Autodesk Inventor part; units mm, degrees
(part 2 of 3)
sketch "Sketch13" plane through (-0.8, 28.2953, 9.6805) normal (0, 0.9365, 0.3507) x (1, 0, 0)
  line L0 (7.3602, 4.8237) -> (7.6197, 4.2211)
  line L1 (7.6197, 4.2211) -> (8.1859, 3.5794)
  line L2 (8.1859, 3.5794) -> (8.8268, 3.0007)
  line L3 (8.8268, 3.0007) -> (9.6093, 2.8387)
  line L4 (9.6093, 2.8387) -> (10.0903, 2.8061)
  line L5 (10.0903, 2.8061) -> (10.4338, 2.9248)
  line L6 (10.4338, 2.9248) -> (11.3689, 4.0829)
  line L7 (11.3689, 4.0829) -> (11.8797, 4.8558)
  line L8 (11.8797, 4.8558) -> (11.9532, 5.0934)
  line L9 (11.9532, 5.0934) -> (11.8798, 5.2528)
  line L10 (11.8798, 5.2528) -> (11.2166, 5.399)
  line L11 (11.2166, 5.399) -> (9.737, 5.4199)
  line L12 (9.737, 5.4199) -> (7.501, 5.3454)
  line L13 (7.501, 5.3454) -> (7.2801, 5.1684)
  line L14 (7.2801, 5.1684) -> (7.3602, 4.8237)
  line L15 (-11.3774, 3.4883) -> (-9.8778, 1.8277)
  line L16 (-9.8778, 1.8277) -> (-9.5845, 1.6866)
  line L17 (-9.5845, 1.6866) -> (-9.3408, 1.793)
  line L18 (-9.3408, 1.793) -> (-8.9771, 2.2117)
  line L19 (-8.9771, 2.2117) -> (-8.6904, 3.7246)
  line L20 (-8.6904, 3.7246) -> (-8.5682, 4.7047)
  line L21 (-8.5682, 4.7047) -> (-8.7396, 5.208)
  line L22 (-8.7396, 5.208) -> (-9.3955, 5.3934)
  line L23 (-9.3955, 5.3934) -> (-10.727, 5.4199)
  line L24 (-10.727, 5.4199) -> (-12.0368, 5.3897)
  line L25 (-12.0368, 5.3897) -> (-12.5412, 5.1784)
  line L26 (-12.5412, 5.1784) -> (-12.301, 4.605)
  line L27 (-12.301, 4.605) -> (-11.3774, 3.4883)
  line L28 (-0.3781, 3.9581) -> (-0.2709, 2.6186)
  line L29 (-0.2709, 2.6186) -> (0.2264, 2.0123)
  line L30 (0.2264, 2.0123) -> (0.7973, 1.6169)
  line L31 (0.7973, 1.6169) -> (1.4201, 1.7538)
  line L32 (1.4201, 1.7538) -> (1.7893, 1.9111)
  line L33 (1.7893, 1.9111) -> (2.0057, 2.1663)
  line L34 (2.0057, 2.1663) -> (2.3158, 3.6997)
  line L35 (2.3158, 3.6997) -> (2.4451, 4.6942)
  line L36 (2.4451, 4.6942) -> (2.3595, 5.2048)
  line L37 (2.3595, 5.2048) -> (1.9431, 5.393)
  line L38 (1.9431, 5.393) -> (1.0799, 5.4199)
  line L39 (1.0799, 5.4199) -> (0.2133, 5.397)
  line L40 (0.2133, 5.397) -> (-0.2274, 5.2372)
  line L41 (-0.2274, 5.2372) -> (-0.379, 4.8032)
  line L42 (-0.379, 4.8032) -> (-0.3781, 3.9581)
  line L43 (-3.9904, 3.904) -> (-3.9296, 3.009)
  line L44 (-3.9296, 3.009) -> (-3.6926, 2.5158)
  line L45 (-3.6926, 2.5158) -> (-3.1853, 2.3017)
  line L46 (-3.1853, 2.3017) -> (-2.3139, 2.2441)
  line L47 (-2.3139, 2.2441) -> (-1.0191, 2.238)
  line L48 (-1.0191, 2.238) -> (-0.6342, 2.358)
  line L49 (-0.6342, 2.358) -> (-0.4353, 2.664)
  line L50 (-0.4353, 2.664) -> (-0.443, 3.9595)
  line L51 (-0.443, 3.9595) -> (-0.4947, 4.8038)
  line L52 (-0.4947, 4.8038) -> (-0.6992, 5.2373)
  line L53 (-0.6992, 5.2373) -> (-1.2249, 5.3971)
  line L54 (-1.2249, 5.3971) -> (-2.2403, 5.4199)
  line L55 (-2.2403, 5.4199) -> (-3.255, 5.3962)
  line L56 (-3.255, 5.3962) -> (-3.7756, 5.2304)
  line L57 (-3.7756, 5.2304) -> (-3.966, 4.7804)
  line L58 (-3.966, 4.7804) -> (-3.9904, 3.904)
  line L59 (-6.7128, 3.5805) -> (-6.6626, 2.522)
  line L60 (-6.6626, 2.522) -> (-6.5055, 2.0099)
  line L61 (-6.5055, 2.0099) -> (-6.1154, 1.9008)
  line L62 (-6.1154, 1.9008) -> (-5.3661, 2.0514)
  line L63 (-5.3661, 2.0514) -> (-4.6053, 2.2664)
  line L64 (-4.6053, 2.2664) -> (-4.2151, 2.5307)
  line L65 (-4.2151, 2.5307) -> (-4.0727, 3.0178)
  line L66 (-4.0727, 3.0178) -> (-4.0552, 3.901)
  line L67 (-4.0552, 3.901) -> (-4.0794, 4.7791)
  line L68 (-4.0794, 4.7791) -> (-4.2288, 5.23)
  line L69 (-4.2288, 5.23) -> (-4.6308, 5.3961)
  line L70 (-4.6308, 5.3961) -> (-5.4126, 5.4199)
  line L71 (-5.4126, 5.4199) -> (-6.1936, 5.3911)
  line L72 (-6.1936, 5.3911) -> (-6.5893, 5.19)
  line L73 (-6.5893, 5.19) -> (-6.7218, 4.6439)
  line L74 (-6.7218, 4.6439) -> (-6.7128, 3.5805)
  line L75 (-7.9017, 1.7773) -> (-7.0187, 1.5649)
  line L76 (-7.0187, 1.5649) -> (-6.8152, 1.6168)
  line L77 (-6.8152, 1.6168) -> (-6.7773, 3.5664)
  line L78 (-6.7773, 3.5664) -> (-6.9182, 5.1882)
  line L79 (-6.9182, 5.1882) -> (-7.1497, 5.3909)
  line L80 (-7.1497, 5.3909) -> (-7.5903, 5.4199)
  line L81 (-7.5903, 5.4199) -> (-8.0343, 5.3934)
  line L82 (-8.0343, 5.3934) -> (-8.29, 5.2082)
  line L83 (-8.29, 5.2082) -> (-8.6244, 3.7268)
  line L84 (-8.6244, 3.7268) -> (-8.767, 2.744)
  line L85 (-8.767, 2.744) -> (-8.7392, 2.2133)
  line L86 (-8.7392, 2.2133) -> (-8.4734, 1.952)
  line L87 (-8.4734, 1.952) -> (-7.9017, 1.7773)
  line L88 (3.0749, 1.6173) -> (3.6583, 1.4472)
  line L89 (3.6583, 1.4472) -> (4.0316, 1.578)
  line L90 (4.0316, 1.578) -> (4.2858, 2.1631)
  line L91 (4.2858, 2.1631) -> (4.5115, 3.356)
  line L92 (4.5115, 3.356) -> (4.6807, 4.5492)
  line L93 (4.6807, 4.5492) -> (4.6567, 5.1618)
  line L94 (4.6567, 5.1618) -> (4.3671, 5.3876)
  line L95 (4.3671, 5.3876) -> (3.7397, 5.4199)
  line L96 (3.7397, 5.4199) -> (3.1031, 5.393)
  line L97 (3.1031, 5.393) -> (2.7493, 5.2047)
  line L98 (2.7493, 5.2047) -> (2.5512, 4.6935)
  line L99 (2.5512, 4.6935) -> (2.3812, 3.6982)
  line L100 (2.3812, 3.6982) -> (2.2432, 2.6972)
  line L101 (2.2432, 2.6972) -> (2.2695, 2.1468)
  line L102 (2.2695, 2.1468) -> (2.5251, 1.8519)
  line L103 (2.5251, 1.8519) -> (3.0749, 1.6173)
  line L104 (10.855, 2.0445) -> (11.1037, 1.6572)
  line L105 (11.1037, 1.6572) -> (11.3976, 1.442)
  line L106 (11.3976, 1.442) -> (12.8812, 1.2175)
  line L107 (12.8812, 1.2175) -> (13.8296, 1.1582)
  line L108 (13.8296, 1.1582) -> (14.3166, 1.3489)
  line L109 (14.3166, 1.3489) -> (14.4961, 1.979)
  line L110 (14.4961, 1.979) -> (14.5216, 3.2379)
  line L111 (14.5216, 3.2379) -> (14.5051, 4.4994)
  line L112 (14.5051, 4.4994) -> (14.3892, 5.1471)
  line L113 (14.3892, 5.1471) -> (14.0745, 5.3858)
  line L114 (14.0745, 5.3858) -> (13.4617, 5.4199)
  line L115 (13.4617, 5.4199) -> (12.8338, 5.3987)
  line L116 (12.8338, 5.3987) -> (12.4135, 5.2505)
  line L117 (12.4135, 5.2505) -> (11.4355, 4.0649)
  line L118 (11.4355, 4.0649) -> (10.6382, 2.7962)
  line L119 (10.6382, 2.7962) -> (10.6471, 2.4504)
  line L120 (10.6471, 2.4504) -> (10.855, 2.0445)
  line L121 (4.6758, 1.0174) -> (5.1233, 0.8083)
  line L122 (5.1233, 0.8083) -> (5.7199, 0.9283)
  line L123 (5.7199, 0.9283) -> (6.0883, 1.0536)
  line L124 (6.0883, 1.0536) -> (6.3365, 1.2754)
  line L125 (6.3365, 1.2754) -> (6.9237, 2.6568)
  line L126 (6.9237, 2.6568) -> (7.4068, 4.0919)
  line L127 (7.4068, 4.0919) -> (7.2944, 4.8155)
  line L128 (7.2944, 4.8155) -> (6.973, 5.3445)
  line L129 (6.973, 5.3445) -> (5.9911, 5.42)
  line L130 (5.9911, 5.42) -> (5.3548, 5.3876)
  line L131 (5.3548, 5.3876) -> (4.9953, 5.1612)
  line L132 (4.9953, 5.1612) -> (4.78, 4.5469)
  line L133 (4.78, 4.5469) -> (4.5762, 3.3505)
  line L134 (4.5762, 3.3505) -> (4.3463, 1.5069)
  line L135 (4.3463, 1.5069) -> (4.4364, 1.2022)
  line L136 (4.4364, 1.2022) -> (4.6758, 1.0174)
  line L137 (-14.1115, 1.6848) -> (-12.9443, 1.2068)
  line L138 (-12.9443, 1.2068) -> (-11.4484, 1.1694)
  line L139 (-11.4484, 1.1694) -> (-10.083, 1.2199)
  line L140 (-10.083, 1.2199) -> (-9.8297, 1.3572)
  line L141 (-9.8297, 1.3572) -> (-9.9803, 1.7344)
  line L142 (-9.9803, 1.7344) -> (-11.4423, 3.4644)
  line L143 (-11.4423, 3.4644) -> (-13.0442, 5.1754)
  line L144 (-13.0442, 5.1754) -> (-13.5398, 5.3893)
  line L145 (-13.5398, 5.3893) -> (-14.1734, 5.4199)
  line L146 (-14.1734, 5.4199) -> (-14.7806, 5.395)
  line L147 (-14.7806, 5.395) -> (-15.0925, 5.2209)
  line L148 (-15.0925, 5.2209) -> (-15.2074, 4.7483)
  line L149 (-15.2074, 4.7483) -> (-15.2238, 3.8281)
  line L150 (-15.2238, 3.8281) -> (-15.2064, 2.8992)
  line L151 (-15.2064, 2.8992) -> (-15.0848, 2.3663)
  line L152 (-15.0848, 2.3663) -> (-14.7545, 2.0285)
  line L153 (-14.7545, 2.0285) -> (-14.1115, 1.6848)
  line L154 (7.2651, 0.6178) -> (8.0505, 0.225)
  line L155 (8.0505, 0.225) -> (8.3951, 0.3155)
  line L156 (8.3951, 0.3155) -> (8.6379, 0.6153)
  line L157 (8.6379, 0.6153) -> (8.7106, 1.6873)
  line L158 (8.7106, 1.6873) -> (8.6743, 2.8168)
  line L159 (8.6743, 2.8168) -> (8.1537, 3.5192)
  line L160 (8.1537, 3.5192) -> (7.7972, 3.8603)
  line L161 (7.7972, 3.8603) -> (7.556, 3.8804)
  line L162 (7.556, 3.8804) -> (6.9793, 2.6209)
  line L163 (6.9793, 2.6209) -> (6.6614, 1.7292)
  line L164 (6.6614, 1.7292) -> (6.5851, 1.2233)
  line L165 (6.5851, 1.2233) -> (6.7775, 0.9154)
  line L166 (6.7775, 0.9154) -> (7.2651, 0.6178)
  line L167 (9.397, 0.394) -> (10.0493, 0.3711)
  line L168 (10.0493, 0.3711) -> (10.6214, 0.8232)
  line L169 (10.6214, 0.8232) -> (11.0623, 1.3709)
  line L170 (11.0623, 1.3709) -> (10.7956, 2.0179)
  line L171 (10.7956, 2.0179) -> (10.3594, 2.61)
  line L172 (10.3594, 2.61) -> (9.6149, 2.7728)
  line L173 (9.6149, 2.7728) -> (9.1541, 2.8072)
  line L174 (9.1541, 2.8072) -> (8.913, 2.7048)
  line L175 (8.913, 2.7048) -> (8.7752, 1.6801)
  line L176 (8.7752, 1.6801) -> (8.8201, 0.6313)
  line L177 (8.8201, 0.6313) -> (9.0129, 0.4715)
  line L178 (9.0129, 0.4715) -> (9.397, 0.394)
  line L179 (-2.9839, 1.2207) -> (-2.3307, 0.3606)
  line L180 (-2.3307, 0.3606) -> (-2.0774, 0.2471)
  line L181 (-2.0774, 0.2471) -> (-1.8529, 0.3751)
  line L182 (-1.8529, 0.3751) -> (-1.4011, 1.2055)
  line L183 (-1.4011, 1.2055) -> (-1.1398, 1.7537)
  line L184 (-1.1398, 1.7537) -> (-1.1472, 2.0378)
  line L185 (-1.1472, 2.0378) -> (-1.5081, 2.1492)
  line L186 (-1.5081, 2.1492) -> (-2.3076, 2.1792)
  line L187 (-2.3076, 2.1792) -> (-3.1035, 2.1789)
  line L188 (-3.1035, 2.1789) -> (-3.4392, 2.079)
  line L189 (-3.4392, 2.079) -> (-3.3782, 1.7896)
  line L190 (-3.3782, 1.7896) -> (-2.9839, 1.2207)
  line L191 (-6.7308, 0.527) -> (-6.6376, -0.0168)
  line L192 (-6.6376, -0.0168) -> (-6.4844, -0.2682)
  line L193 (-6.4844, -0.2682) -> (-6.168, -0.2879)
  line L194 (-6.168, -0.2879) -> (-5.5853, -0.1364)
  line L195 (-5.5853, -0.1364) -> (-4.6798, 0.2502)
  line L196 (-4.6798, 0.2502) -> (-4.3418, 1.2207)
  line L197 (-4.3418, 1.2207) -> (-4.2212, 1.8332)
  line L198 (-4.2212, 1.8332) -> (-4.2898, 2.1165)
  line L199 (-4.2898, 2.1165) -> (-4.6457, 2.1416)
  line L200 (-4.6457, 2.1416) -> (-5.3868, 1.9798)
  line L201 (-5.3868, 1.9798) -> (-6.768, 1.5724)
  line L202 (-6.768, 1.5724) -> (-6.7308, 0.527)
  line L203 (-1.0882, -0.3506) -> (-0.6512, -0.6727)
  line L204 (-0.6512, -0.6727) -> (-0.3715, -0.7289)
  line L205 (-0.3715, -0.7289) -> (-0.1283, -0.4729)
  line L206 (-0.1283, -0.4729) -> (0.199, 0.1411)
  line L207 (0.199, 0.1411) -> (0.6103, 1.37)
  line L208 (0.6103, 1.37) -> (0.5042, 1.6593)
  line L209 (0.5042, 1.6593) -> (0.189, 1.959)
  line L210 (0.189, 1.959) -> (-0.3301, 2.3635)
  line L211 (-0.3301, 2.3635) -> (-0.6027, 2.3013)
  line L212 (-0.6027, 2.3013) -> (-0.8674, 2.0585)
  line L213 (-0.8674, 2.0585) -> (-1.3318, 1.1985)
  line L214 (-1.3318, 1.1985) -> (-1.6745, 0.2827)
  line L215 (-1.6745, 0.2827) -> (-1.5089, 0.0034)
  line L216 (-1.5089, 0.0034) -> (-1.0882, -0.3506)
  line L217 (1.6614, 0.2868) -> (2.165, -0.2401)
  line L218 (2.165, -0.2401) -> (2.4979, -0.4164)
  line L219 (2.4979, -0.4164) -> (2.8085, -0.2428)
  line L220 (2.8085, -0.2428) -> (3.2452, 0.28)
  line L221 (3.2452, 0.28) -> (3.6539, 0.823)
  line L222 (3.6539, 0.823) -> (3.7676, 1.1381)
  line L223 (3.7676, 1.1381) -> (3.5661, 1.3453)
  line L224 (3.5661, 1.3453) -> (3.0291, 1.5654)
  line L225 (3.0291, 1.5654) -> (2.1198, 1.8482)
  line L226 (2.1198, 1.8482) -> (1.4471, 1.6946)
  line L227 (1.4471, 1.6946) -> (1.0921, 1.4076)
  line L228 (1.0921, 1.4076) -> (0.996, 1.1652)
  line L229 (0.996, 1.1652) -> (1.6614, 0.2868)
  line L230 (-9.7711, 0.2547) -> (-9.6535, -0.5893)
  line L231 (-9.6535, -0.5893) -> (-9.264, -1.019)
  line L232 (-9.264, -1.019) -> (-8.6109, -1.3907)
  line L233 (-8.6109, -1.3907) -> (-7.5291, -0.9139)
  line L234 (-7.5291, -0.9139) -> (-6.7895, -0.3691)
  line L235 (-6.7895, -0.3691) -> (-6.7948, 0.5164)
  line L236 (-6.7948, 0.5164) -> (-7.0333, 1.3732)
  line L237 (-7.0333, 1.3732) -> (-7.9267, 1.7168)
  line L238 (-7.9267, 1.7168) -> (-8.852, 1.9124)
  line L239 (-8.852, 1.9124) -> (-9.3137, 1.7335)
  line L240 (-9.3137, 1.7335) -> (-9.7708, 1.33)
  line L241 (-9.7708, 1.33) -> (-9.7711, 0.2547)
  line L242 (-9.7711, 0.2547) -> (-9.7711, 0.2547)
  line L243 (-3.9817, -0.3783) -> (-3.4389, -0.7611)
  line L244 (-3.4389, -0.7611) -> (-2.8819, -0.3441)
  line L245 (-2.8819, -0.3441) -> (-2.57, -0.0103)
  line L246 (-2.57, -0.0103) -> (-2.4841, 0.2629)
  line L247 (-2.4841, 0.2629) -> (-3.0563, 1.21)
  line L248 (-3.0563, 1.21) -> (-3.6206, 1.8321)
  line L249 (-3.6206, 1.8321) -> (-3.9356, 2.0413)
  line L250 (-3.9356, 2.0413) -> (-4.1153, 1.8389)
  line L251 (-4.1153, 1.8389) -> (-4.274, 1.2267)
  line L252 (-4.274, 1.2267) -> (-4.4236, 0.2094)
  line L253 (-4.4236, 0.2094) -> (-3.9817, -0.3783)
  line L254 (-12.1877, -0.0457) -> (-11.42, -0.9898)
  line L255 (-11.42, -0.9898) -> (-11.0899, -1.0362)
  line L256 (-11.0899, -1.0362) -> (-10.5968, -0.9062)
  line L257 (-10.5968, -0.9062) -> (-9.8774, -0.5711)
  line L258 (-9.8774, -0.5711) -> (-9.8354, 0.2446)
  line L259 (-9.8354, 0.2446) -> (-9.9001, 0.7619)
  line L260 (-9.9001, 0.7619) -> (-10.0874, 1.024)
  line L261 (-10.0874, 1.024) -> (-11.4262, 1.1051)
  line L262 (-11.4262, 1.1051) -> (-12.293, 1.0672)
  line L263 (-12.293, 1.0672) -> (-12.6613, 0.9348)
  line L264 (-12.6613, 0.9348) -> (-12.6024, 0.5997)
  line L265 (-12.6024, 0.5997) -> (-12.1877, -0.0457)
  line L266 (10.4088, -0.4645) -> (10.6102, -0.8723)
  line L267 (10.6102, -0.8723) -> (10.907, -1.0492)
  line L268 (10.907, -1.0492) -> (12.6137, -0.8583)
  line L269 (12.6137, -0.8583) -> (14.2832, -0.4825)
  line L270 (14.2832, -0.4825) -> (14.4919, -0.2206)
  line L271 (14.4919, -0.2206) -> (14.5217, 0.2264)
  line L272 (14.5217, 0.2264) -> (14.496, 0.6709)
  line L273 (14.496, 0.6709) -> (14.3161, 0.9155)
  line L274 (14.3161, 0.9155) -> (12.8772, 1.1528)
  line L275 (12.8772, 1.1528) -> (11.3682, 1.2279)
  line L276 (11.3682, 1.2279) -> (11.0219, 1.0874)
  line L277 (11.0219, 1.0874) -> (10.6723, 0.782)
  line L278 (10.6723, 0.782) -> (10.2191, 0.2267)
  line L279 (10.2191, 0.2267) -> (10.4088, -0.4645)
  line L280 (0.2521, -1.4362) -> (0.8238, -1.7459)
  line L281 (0.8238, -1.7459) -> (1.5876, -1.6747)
  line L282 (1.5876, -1.6747) -> (2.29, -1.5051)
  line L283 (2.29, -1.5051) -> (2.432, -1.1254)
  line L284 (2.432, -1.1254) -> (2.3686, -0.6459)
  line L285 (2.3686, -0.6459) -> (1.6328, 0.2219)
  line L286 (1.6328, 0.2219) -> (1.1342, 0.7443)
  line L287 (1.1342, 0.7443) -> (0.8231, 0.9038)
  line L288 (0.8231, 0.9038) -> (0.569, 0.6872)
  line L289 (0.569, 0.6872) -> (0.2415, 0.0815)
  line L290 (0.2415, 0.0815) -> (-0.1541, -0.9666)
  line L291 (-0.1541, -0.9666) -> (-0.0517, -1.2026)
  line L292 (-0.0517, -1.2026) -> (0.2521, -1.4362)
  line L293 (5.216, -0.2767) -> (5.4184, -1.1695)
  line L294 (5.4184, -1.1695) -> (6.3084, -1.5912)
  line L295 (6.3084, -1.5912) -> (7.2128, -1.8804)
  line L296 (7.2128, -1.8804) -> (7.5157, -1.8465)
  line L297 (7.5157, -1.8465) -> (7.7162, -1.6541)
  line L298 (7.7162, -1.6541) -> (7.9036, -0.8344)
  line L299 (7.9036, -0.8344) -> (7.9576, 0.0338)
  line L300 (7.9576, 0.0338) -> (7.2253, 0.5657)
  line L301 (7.2253, 0.5657) -> (6.3928, 0.9604)
  line L302 (6.3928, 0.9604) -> (5.7451, 0.8681)
  line L303 (5.7451, 0.8681) -> (5.2162, 0.5948)
  line L304 (5.2162, 0.5948) -> (5.216, -0.2767)
  line L305 (2.5874, -1.6757) -> (3.6223, -1.8508)
  line L306 (3.6223, -1.8508) -> (4.4502, -1.8576)
  line L307 (4.4502, -1.8576) -> (4.8783, -1.5817)
  line L308 (4.8783, -1.5817) -> (5.1835, -1.1766)
  line L309 (5.1835, -1.1766) -> (5.1512, -0.2796)
  line L310 (5.1512, -0.2796) -> (5.0205, 0.6103)
  line L311 (5.0205, 0.6103) -> (4.6372, 0.9651)
  line L312 (4.6372, 0.9651) -> (4.2853, 1.0833)
  line L313 (4.2853, 1.0833) -> (4.0285, 1.0473)
  line L314 (4.0285, 1.0473) -> (3.2973, 0.2413)
  line L315 (3.2973, 0.2413) -> (2.6334, -0.646)
  line L316 (2.6334, -0.646) -> (2.4963, -1.1337)
  line L317 (2.4963, -1.1337) -> (2.4707, -1.5172)
  line L318 (2.4707, -1.5172) -> (2.5874, -1.6757)
  line L319 (-13.7731, -2.0728) -> (-12.4514, -2.1523)
  line L320 (-12.4514, -2.1523) -> (-12.1681, -2.016)
  line L321 (-12.1681, -2.016) -> (-11.9027, -1.7178)
  line L322 (-11.9027, -1.7178) -> (-11.6721, -1.3992)
  line L323 (-11.6721, -1.3992) -> (-11.632, -1.1205)
  line L324 (-11.632, -1.1205) -> (-12.2556, -0.061)
  line L325 (-12.2556, -0.061) -> (-13.069, 1.0015)
  line L326 (-13.069, 1.0015) -> (-14.1261, 1.6197)
  line L327 (-14.1261, 1.6197) -> (-14.7607, 1.9025)
  line L328 (-14.7607, 1.9025) -> (-15.0866, 1.8414)
  line L329 (-15.0866, 1.8414) -> (-15.2067, 1.2966)
  line L330 (-15.2067, 1.2966) -> (-15.2238, 0.1282)
  line L331 (-15.2238, 0.1282) -> (-15.2011, -1.0513)
  line L332 (-15.2011, -1.0513) -> (-15.0425, -1.6737)
  line L333 (-15.0425, -1.6737) -> (-14.6118, -1.9454)
  line L334 (-14.6118, -1.9454) -> (-13.7731, -2.0728)
  line L335 (8.8189, -2.3255) -> (9.4326, -2.6307)
  line L336 (9.4326, -2.6307) -> (9.8007, -2.694)
  line L337 (9.8007, -2.694) -> (10.0437, -2.4991)
  line L338 (10.0437, -2.4991) -> (10.2821, -2.0299)
  line L339 (10.2821, -2.0299) -> (10.5668, -1.2259)
  line L340 (10.5668, -1.2259) -> (10.3504, -0.493)
  line L341 (10.3504, -0.493) -> (10.0039, 0.151)
  line L342 (10.0039, 0.151) -> (9.3778, 0.3313)
  line L343 (9.3778, 0.3313) -> (8.7547, 0.3999)
  line L344 (8.7547, 0.3999) -> (8.4296, 0.2606)
  line L345 (8.4296, 0.2606) -> (8.1654, -0.0072)
  line L346 (8.1654, -0.0072) -> (7.9688, -0.8389)
  line L347 (7.9688, -0.8389) -> (7.8778, -1.3828)
  line L348 (7.8778, -1.3828) -> (7.936, -1.7189)
  line L349 (7.936, -1.7189) -> (8.8189, -2.3255)
  line L350 (-5.5732, -1.7792) -> (-4.6622, -2.8963)
  line L351 (-4.6622, -2.8963) -> (-4.3883, -2.9878)
  line L352 (-4.3883, -2.9878) -> (-4.0445, -2.9091)
  line L353 (-4.0445, -2.9091) -> (-3.5467, -2.6476)
  line L354 (-3.5467, -2.6476) -> (-3.4746, -1.8455)
  line L355 (-3.4746, -1.8455) -> (-3.5419, -0.9996)
  line L356 (-3.5419, -0.9996) -> (-4.0201, -0.4313)
  line L357 (-4.0201, -0.4313) -> (-4.6213, -0.01)
  line L358 (-4.6213, -0.01) -> (-5.55, -0.1936)
  line L359 (-5.55, -0.1936) -> (-6.1034, -0.3783)
  line L360 (-6.1034, -0.3783) -> (-6.2903, -0.6051)
  line L361 (-6.2903, -0.6051) -> (-6.1128, -1.0225)
  line L362 (-6.1128, -1.0225) -> (-5.5732, -1.7792)
  line L363 (-2.7913, -2.702) -> (-2.1549, -2.5615)
  line L364 (-2.1549, -2.5615) -> (-1.274, -1.8624)
  line L365 (-1.274, -1.8624) -> (-0.7606, -1.3573)
  line L366 (-0.7606, -1.3573) -> (-0.5738, -1.0372)
  line L367 (-0.5738, -1.0372) -> (-0.6994, -0.7655)
  line L368 (-0.6994, -0.7655) -> (-1.1232, -0.4056)
  line L369 (-1.1232, -0.4056) -> (-1.8102, 0.1174)
  line L370 (-1.8102, 0.1174) -> (-2.0733, 0.1824)
  line L371 (-2.0733, 0.1824) -> (-2.3131, 0.1022)
  line L372 (-2.3131, 0.1022) -> (-2.8372, -0.391)
  line L373 (-2.8372, -0.391) -> (-3.3373, -0.9945)
  line L374 (-3.3373, -0.9945) -> (-3.4098, -1.8464)
  line L375 (-3.4098, -1.8464) -> (-3.3153, -2.6306)
  line L376 (-3.3153, -2.6306) -> (-2.7913, -2.702)
  line L377 (11.8788, -3.0384) -> (13.5806, -3.1991)
  line L378 (13.5806, -3.1991) -> (14.1459, -3.1309)
  line L379 (14.1459, -3.1309) -> (14.3631, -3.0506)
  line L380 (14.3631, -3.0506) -> (14.4747, -2.8867)
  line L381 (14.4747, -2.8867) -> (14.5216, -1.8142)
  line L382 (14.5216, -1.8142) -> (14.4919, -1.1194)
  line L383 (14.4919, -1.1194) -> (14.2833, -0.7951)
  line L384 (14.2833, -0.7951) -> (13.7172, -0.7577)
  line L385 (13.7172, -0.7577) -> (12.6149, -0.9238)
  line L386 (12.6149, -0.9238) -> (10.9013, -1.3035)
  line L387 (10.9013, -1.3035) -> (10.5859, -1.5754)
  line L388 (10.5859, -1.5754) -> (10.3478, -2.0417)
  line L389 (10.3478, -2.0417) -> (10.1692, -2.5061)
  line L390 (10.1692, -2.5061) -> (10.2691, -2.7647)
  line L391 (10.2691, -2.7647) -> (11.8788, -3.0384)
  line L392 (-7.5951, -2.6194) -> (-6.8398, -3.6386)
  line L393 (-6.8398, -3.6386) -> (-6.5112, -3.7495)
  line L394 (-6.5112, -3.7495) -> (-6.0182, -3.734)
  line L395 (-6.0182, -3.734) -> (-5.2574, -3.6477)
  line L396 (-5.2574, -3.6477) -> (-4.9267, -3.3955)
  line L397 (-4.9267, -3.3955) -> (-4.7922, -3.2132)
  line L398 (-4.7922, -3.2132) -> (-4.8214, -2.9864)
  line L399 (-4.8214, -2.9864) -> (-5.6375, -1.8012)
  line L400 (-5.6375, -1.8012) -> (-6.2233, -1.0443)
  line L401 (-6.2233, -1.0443) -> (-6.6108, -0.7047)
  line L402 (-6.6108, -0.7047) -> (-6.9732, -0.7037)
  line L403 (-6.9732, -0.7037) -> (-7.4835, -0.9626)
  line L404 (-7.4835, -0.9626) -> (-7.9666, -1.2605)
  line L405 (-7.9666, -1.2605) -> (-8.1393, -1.5324)
  line L406 (-8.1393, -1.5324) -> (-8.012, -1.9336)
  line L407 (-8.012, -1.9336) -> (-7.5951, -2.6194)
  line L408 (-11.9751, -2.8425) -> (-11.5966, -3.3367)
  line L409 (-11.5966, -3.3367) -> (-10.7155, -3.3983)
  line L410 (-10.7155, -3.3983) -> (-9.8168, -3.2661)
  line L411 (-9.8168, -3.2661) -> (-9.3158, -2.4042)
  line L412 (-9.3158, -2.4042) -> (-8.9889, -1.4992)
  line L413 (-8.9889, -1.4992) -> (-9.0684, -1.2862)
  line L414 (-9.0684, -1.2862) -> (-9.3092, -1.0657)
  line L415 (-9.3092, -1.0657) -> (-9.7892, -0.7874)
  line L416 (-9.7892, -0.7874) -> (-10.5805, -0.969)
  line L417 (-10.5805, -0.969) -> (-11.3711, -1.2605)
  line L418 (-11.3711, -1.2605) -> (-11.8468, -1.7517)
  line L419 (-11.8468, -1.7517) -> (-12.1802, -2.2813)
  line L420 (-12.1802, -2.2813) -> (-11.9751, -2.8425)
  line L421 (4.8263, -3.3054) -> (5.0747, -4.5083)
  line L422 (5.0747, -4.5083) -> (5.2376, -4.7949)
  line L423 (5.2376, -4.7949) -> (5.4307, -4.8933)
  line L424 (5.4307, -4.8933) -> (5.833, -4.76)
  line L425 (5.833, -4.76) -> (6.2781, -4.4471)
  line L426 (6.2781, -4.4471) -> (6.7712, -3.2885)
  line L427 (6.7712, -3.2885) -> (7.0454, -2.5318)
  line L428 (7.0454, -2.5318) -> (7.0851, -2.1087)
  line L429 (7.0851, -2.1087) -> (6.8443, -1.8656)
  line L430 (6.8443, -1.8656) -> (6.2765, -1.6487)
  line L431 (6.2765, -1.6487) -> (5.3605, -1.3913)
  line L432 (5.3605, -1.3913) -> (4.9223, -1.6292)
  line L433 (4.9223, -1.6292) -> (4.719, -1.8357)
  line L434 (4.719, -1.8357) -> (4.6413, -2.0792)
  line L435 (4.6413, -2.0792) -> (4.8263, -3.3054)
  line L436 (-1.3768, -3.3141) -> (-0.648, -3.8496)
  line L437 (-0.648, -3.8496) -> (-0.0792, -3.8271)
  line L438 (-0.0792, -3.8271) -> (0.4129, -3.6103)
  line L439 (0.4129, -3.6103) -> (0.6059, -2.7851)
  line L440 (0.6059, -2.7851) -> (0.6647, -1.9285)
  line L441 (0.6647, -1.9285) -> (0.2172, -1.4909)
  line L442 (0.2172, -1.4909) -> (-0.1045, -1.2905)
  line L443 (-0.1045, -1.2905) -> (-0.3618, -1.2668)
  line L444 (-0.3618, -1.2668) -> (-1.2235, -1.9044)
  line L445 (-1.2235, -1.9044) -> (-1.7371, -2.3659)
  line L446 (-1.7371, -2.3659) -> (-1.9243, -2.6666)
  line L447 (-1.9243, -2.6666) -> (-1.7994, -2.9386)
  line L448 (-1.7994, -2.9386) -> (-1.3768, -3.3141)
  line L449 (0.9761, -4.1392) -> (1.6739, -4.5976)
  line L450 (1.6739, -4.5976) -> (1.9368, -4.6091)
  line L451 (1.9368, -4.6091) -> (2.2901, -4.4139)
  line L452 (2.2901, -4.4139) -> (2.6139, -4.0667)
  line L453 (2.6139, -4.0667) -> (2.6704, -3.0137)
  line L454 (2.6704, -3.0137) -> (2.6635, -1.9743)
  line L455 (2.6635, -1.9743) -> (2.5428, -1.7227)
  line L456 (2.5428, -1.7227) -> (2.3212, -1.6343)
  line L457 (2.3212, -1.6343) -> (1.6079, -1.737)
  line L458 (1.6079, -1.737) -> (0.8942, -1.9707)
  line L459 (0.8942, -1.9707) -> (0.6694, -2.7991)
  line L460 (0.6694, -2.7991) -> (0.6003, -3.6623)
  line L461 (0.6003, -3.6623) -> (0.9761, -4.1392)
  line L462 (3.8707, -4.4062) -> (4.5301, -4.5185)
  line L463 (4.5301, -4.5185) -> (4.8425, -4.441)
  line L464 (4.8425, -4.441) -> (4.8913, -4.0702)
  line L465 (4.8913, -4.0702) -> (4.7597, -3.3026)
  line L466 (4.7597, -3.3026) -> (4.4239, -2.1288)
  line L467 (4.4239, -2.1288) -> (4.1353, -1.9672)
  line L468 (4.1353, -1.9672) -> (3.6241, -1.9158)
  line L469 (3.6241, -1.9158) -> (3.1169, -1.9033)
  line L470 (3.1169, -1.9033) -> (2.8552, -2.014)
  line L471 (2.8552, -2.014) -> (2.7352, -3.0194)
  line L472 (2.7352, -3.0194) -> (2.7462, -3.6916)
  line L473 (2.7462, -3.6916) -> (2.8682, -4.0601)
  line L474 (2.8682, -4.0601) -> (3.2076, -4.255)
  line L475 (3.2076, -4.255) -> (3.8707, -4.4062)
  line L476 (-9.4981, -3.8379) -> (-9.2124, -4.2134)
  line L477 (-9.2124, -4.2134) -> (-8.3857, -4.331)
  line L478 (-8.3857, -4.331) -> (-7.5485, -4.3598)
  line L479 (-7.5485, -4.3598) -> (-7.1889, -4.1139)
  line L480 (-7.1889, -4.1139) -> (-7.0386, -3.9268)
  line L481 (-7.0386, -3.9268) -> (-7.0372, -3.7114)
  line L482 (-7.0372, -3.7114) -> (-7.6561, -2.6442)
  line L483 (-7.6561, -2.6442) -> (-8.3361, -1.6121)
  line L484 (-8.3361, -1.6121) -> (-8.6121, -1.4555)
  line L485 (-8.6121, -1.4555) -> (-8.8493, -1.5696)
  line L486 (-8.8493, -1.5696) -> (-9.2573, -2.4322)
  line L487 (-9.2573, -2.4322) -> (-9.6148, -3.3484)
  line L488 (-9.6148, -3.3484) -> (-9.4981, -3.8379)
  line L489 (7.2856, -4.8632) -> (7.8457, -5.0033)
  line L490 (7.8457, -5.0033) -> (8.2136, -4.9656)
  line L491 (8.2136, -4.9656) -> (9.0253, -4.0529)
  line L492 (9.0253, -4.0529) -> (9.4694, -3.4021)
  line L493 (9.4694, -3.4021) -> (9.5922, -3.0109)
  line L494 (9.5922, -3.0109) -> (9.3711, -2.7225)
  line L495 (9.3711, -2.7225) -> (8.7834, -2.38)
  line L496 (8.7834, -2.38) -> (7.8497, -1.8989)
  line L497 (7.8497, -1.8989) -> (7.5426, -1.9055)
  line L498 (7.5426, -1.9055) -> (7.3026, -2.1447)
  line L499 (7.3026, -2.1447) -> (6.839, -3.2924)
  line L500 (6.839, -3.2924) -> (6.5643, -4.0477)
  line L501 (6.5643, -4.0477) -> (6.5192, -4.4631)
  line L502 (6.5192, -4.4631) -> (6.7457, -4.6858)
  line L503 (6.7457, -4.6858) -> (7.2856, -4.8632)
  line L504 (-13.7646, -5.5678) -> (-12.9165, -5.5166)
  line L505 (-12.9165, -5.5166) -> (-12.4521, -5.3858)
  line L506 (-12.4521, -5.3858) -> (-12.2078, -5.0731)
  line L507 (-12.2078, -5.0731) -> (-12.02, -4.4761)
  line L508 (-12.02, -4.4761) -> (-11.8074, -3.5026)
  line L509 (-11.8074, -3.5026) -> (-12.0319, -2.8738)
  line L510 (-12.0319, -2.8738) -> (-12.2264, -2.5409)
  line L511 (-12.2264, -2.5409) -> (-12.473, -2.3533)
  line L512 (-12.473, -2.3533) -> (-13.7765, -2.1376)
  line L513 (-13.7765, -2.1376) -> (-14.6132, -2.0709)
  line L514 (-14.6132, -2.0709) -> (-15.0429, -2.2218)
  line L515 (-15.0429, -2.2218) -> (-15.2012, -2.7465)
  line L516 (-15.2012, -2.7465) -> (-15.2238, -3.8006)
  line L517 (-15.2238, -3.8006) -> (-15.201, -4.8564)
  line L518 (-15.201, -4.8564) -> (-15.0414, -5.3924)
  line L519 (-15.0414, -5.3924) -> (-14.6082, -5.5743)
  line L520 (-14.6082, -5.5743) -> (-13.7646, -5.5678)
  line L521 (10.5394, -4.1975) -> (10.9515, -4.887)
  line L522 (10.9515, -4.887) -> (11.308, -5.1345)
  line L523 (11.308, -5.1345) -> (11.7675, -4.9537)
  line L524 (11.7675, -4.9537) -> (12.489, -4.3584)
  line L525 (12.489, -4.3584) -> (13.1575, -3.7403)
  line L526 (13.1575, -3.7403) -> (13.3109, -3.403)
  line L527 (13.3109, -3.403) -> (12.8866, -3.2281)
  line L528 (12.8866, -3.2281) -> (11.8221, -3.0976)
  line L529 (11.8221, -3.0976) -> (10.7109, -3.0471)
  line L530 (10.7109, -3.0471) -> (10.2069, -3.1449)
  line L531 (10.2069, -3.1449) -> (10.1898, -3.494)
  line L532 (10.1898, -3.494) -> (10.5394, -4.1975)
  line L533 (-2.8671, -4.1264) -> (-2.3658, -5.2555)
  line L534 (-2.3658, -5.2555) -> (-2.1195, -5.3481)
  line L535 (-2.1195, -5.3481) -> (-1.7346, -5.2687)
  line L536 (-1.7346, -5.2687) -> (-1.1375, -5.0482)
  line L537 (-1.1375, -5.0482) -> (-0.875, -4.5418)
  line L538 (-0.875, -4.5418) -> (-0.7895, -3.9777)
  line L539 (-0.7895, -3.9777) -> (-1.4307, -3.3536)
  line L540 (-1.4307, -3.3536) -> (-2.1699, -2.8045)
  line L541 (-2.1699, -2.8045) -> (-2.7699, -2.7653)
  line L542 (-2.7699, -2.7653) -> (-3.0959, -2.8124)
  line L543 (-3.0959, -2.8124) -> (-3.2147, -2.9698)
  line L544 (-3.2147, -2.9698) -> (-2.8671, -4.1264)
  line L545 (-11.0081, -5.4507) -> (-9.9274, -5.295)
  line L546 (-9.9274, -5.295) -> (-9.5821, -4.8182)
  line L547 (-9.5821, -4.8182) -> (-9.4116, -4.3019)
  line L548 (-9.4116, -4.3019) -> (-9.5546, -3.8702)
  line L549 (-9.5546, -3.8702) -> (-9.8458, -3.5061)
  line L550 (-9.8458, -3.5061) -> (-10.7125, -3.4631)
  line L551 (-10.7125, -3.4631) -> (-11.2735, -3.4852)
  line L552 (-11.2735, -3.4852) -> (-11.5904, -3.6006)
  line L553 (-11.5904, -3.6006) -> (-11.9594, -4.5001)
  line L554 (-11.9594, -4.5001) -> (-12.0862, -5.1071)
  line L555 (-12.0862, -5.1071) -> (-12.0294, -5.4084)
  line L556 (-12.0294, -5.4084) -> (-11.6998, -5.4933)
  line L557 (-11.6998, -5.4933) -> (-11.0081, -5.4507)
  line L558 (8.3945, -5.3923) -> (8.5859, -5.6294)
  line L559 (8.5859, -5.6294) -> (9.2607, -5.9861)
  line L560 (9.2607, -5.9861) -> (9.9917, -6.2581)
  line L561 (9.9917, -6.2581) -> (10.5758, -5.9019)
  line L562 (10.5758, -5.9019) -> (10.8893, -5.6167)
  line L563 (10.8893, -5.6167) -> (10.9849, -5.3488)
  line L564 (10.9849, -5.3488) -> (10.4901, -4.2425)
  line L565 (10.4901, -4.2425) -> (10.1047, -3.5663)
  line L566 (10.1047, -3.5663) -> (9.8277, -3.327)
  line L567 (9.8277, -3.327) -> (9.5254, -3.5123)
  line L568 (9.5254, -3.5123) -> (9.0641, -4.1096)
  line L569 (9.0641, -4.1096) -> (8.3951, -5.0692)
  line L570 (8.3951, -5.0692) -> (8.3945, -5.3923)
  line L571 (-0.5382, -5.6484) -> (-0.2485, -5.9438)
  line L572 (-0.2485, -5.9438) -> (-0.0277, -6.0146)
  line L573 (-0.0277, -6.0146) -> (0.6546, -5.3826)
  line L574 (0.6546, -5.3826) -> (1.2215, -4.6334)
  line L575 (1.2215, -4.6334) -> (1.168, -4.4258)
  line L576 (1.168, -4.4258) -> (0.9237, -4.1791)
  line L577 (0.9237, -4.1791) -> (0.4691, -3.8391)
  line L578 (0.4691, -3.8391) -> (-0.062, -3.8897)
  line L579 (-0.062, -3.8897) -> (-0.5637, -4.0604)
  line L580 (-0.5637, -4.0604) -> (-0.8129, -4.5606)
  line L581 (-0.8129, -4.5606) -> (-0.9338, -5.113)
  line L582 (-0.9338, -5.113) -> (-0.5382, -5.6484)
  line L583 (-5.0223, -4.757) -> (-4.8352, -5.7093)
  line L584 (-4.8352, -5.7093) -> (-4.2116, -6.1407)
  line L585 (-4.2116, -6.1407) -> (-3.5568, -6.4238)
  line L586 (-3.5568, -6.4238) -> (-3.1504, -6.3372)
  line L587 (-3.1504, -6.3372) -> (-2.8096, -6.1632)
  line L588 (-2.8096, -6.1632) -> (-2.6142, -5.8339)
  line L589 (-2.6142, -5.8339) -> (-2.5251, -5.3561)
  line L590 (-2.5251, -5.3561) -> (-2.9301, -4.1429)
  line L591 (-2.9301, -4.1429) -> (-3.4532, -2.9863)
  line L592 (-3.4532, -2.9863) -> (-3.6822, -2.8911)
  line L593 (-3.6822, -2.8911) -> (-4.0264, -2.9713)
  line L594 (-4.0264, -2.9713) -> (-4.5684, -3.1603)
  line L595 (-4.5684, -3.1603) -> (-4.8724, -3.4322)
  line L596 (-4.8724, -3.4322) -> (-5.0894, -3.8121)
  line L597 (-5.0894, -3.8121) -> (-5.0223, -4.757)
  line L598 (-9.3664, -6.0112) -> (-8.9415, -6.5736)
  line L599 (-8.9415, -6.5736) -> (-8.2469, -6.7018)
  line L600 (-8.2469, -6.7018) -> (-7.8192, -6.7162)
  line L601 (-7.8192, -6.7162) -> (-7.5986, -6.6076)
  line L602 (-7.5986, -6.6076) -> (-7.4981, -5.6133)
  line L603 (-7.4981, -5.6133) -> (-7.6034, -4.6028)
  line L604 (-7.6034, -4.6028) -> (-7.8717, -4.4557)
  line L605 (-7.8717, -4.4557) -> (-8.396, -4.3952)
  line L606 (-8.396, -4.3952) -> (-9.2174, -4.3965)
  line L607 (-9.2174, -4.3965) -> (-9.5247, -4.8489)
  line L608 (-9.5247, -4.8489) -> (-9.6711, -5.3899)
  line L609 (-9.6711, -5.3899) -> (-9.3664, -6.0112)
  line L610 (-7.1401, -7.0356) -> (-6.9506, -7.173)
  line L611 (-6.9506, -7.173) -> (-6.7588, -7.168)
  line L612 (-6.7588, -7.168) -> (-5.9049, -6.5483)
  line L613 (-5.9049, -6.5483) -> (-5.1031, -5.7674)
  line L614 (-5.1031, -5.7674) -> (-5.0858, -4.7722)
  line L615 (-5.0858, -4.7722) -> (-5.2886, -3.8774)
  line L616 (-5.2886, -3.8774) -> (-5.5464, -3.782)
  line L617 (-5.5464, -3.782) -> (-6.0262, -3.7995)
  line L618 (-6.0262, -3.7995) -> (-6.7854, -3.8876)
  line L619 (-6.7854, -3.8876) -> (-7.1385, -4.155)
  line L620 (-7.1385, -4.155) -> (-7.3894, -4.5605)
  line L621 (-7.3894, -4.5605) -> (-7.4333, -5.615)
  line L622 (-7.4333, -5.615) -> (-7.4037, -6.6646)
  line L623 (-7.4037, -6.6646) -> (-7.1401, -7.0356)
  line L624 (12.9313, -6.893) -> (13.8505, -7.6832)
  line L625 (13.8505, -7.6832) -> (14.3224, -7.8235)
  line L626 (14.3224, -7.8235) -> (14.4963, -7.2031)
  line L627 (14.4963, -7.2031) -> (14.5211, -5.7111)
  line L628 (14.5211, -5.7111) -> (14.4751, -3.4319)
  line L629 (14.4751, -3.4319) -> (14.3663, -3.1762)
  line L630 (14.3663, -3.1762) -> (14.1545, -3.1952)
  line L631 (14.1545, -3.1952) -> (13.6809, -3.4207)
  line L632 (13.6809, -3.4207) -> (12.5647, -4.3772)
  line L633 (12.5647, -4.3772) -> (11.8823, -5.023)
  line L634 (11.8823, -5.023) -> (11.6931, -5.5003)
  line L635 (11.6931, -5.5003) -> (12.0313, -6.0451)
  line L636 (12.0313, -6.0451) -> (12.9313, -6.893)
  line L637 (2.2673, -5.9906) -> (2.4636, -6.7227)
  line L638 (2.4636, -6.7227) -> (2.7038, -6.9805)
  line L639 (2.7038, -6.9805) -> (3.1452, -6.7763)
  line L640 (3.1452, -6.7763) -> (3.9451, -6.1227)
  line L641 (3.9451, -6.1227) -> (5.1313, -5.0871)
  line L642 (5.1313, -5.0871) -> (5.2407, -4.9226)
  line L643 (5.2407, -4.9226) -> (5.1823, -4.8324)
  line L644 (5.1823, -4.8324) -> (3.8705, -4.4723)
  line L645 (3.8705, -4.4723) -> (2.7978, -4.2947)
  line L646 (2.7978, -4.2947) -> (2.3309, -4.4648)
  line L647 (2.3309, -4.4648) -> (2.1241, -4.6169)
  line L648 (2.1241, -4.6169) -> (2.0486, -4.8266)
  line L649 (2.0486, -4.8266) -> (2.2673, -5.9906)
  line L650 (0.0292, -7.3936) -> (0.117, -8.497)
  line L651 (0.117, -8.497) -> (0.4165, -9.3072)
  line L652 (0.4165, -9.3072) -> (0.7707, -9.9733)
  line L653 (0.7707, -9.9733) -> (1.2411, -10.0685)
  line L654 (1.2411, -10.0685) -> (1.5304, -10.0472)
  line L655 (1.5304, -10.0472) -> (1.7187, -9.8983)
  line L656 (1.7187, -9.8983) -> (2.1238, -8.7074)
  line L657 (2.1238, -8.7074) -> (2.4291, -7.3515)
  line L658 (2.4291, -7.3515) -> (2.2091, -6.0261)
  line L659 (2.2091, -6.0261) -> (1.91, -4.8652)
  line L660 (1.91, -4.8652) -> (1.6623, -4.6614)
  line L661 (1.6623, -4.6614) -> (1.3626, -4.7241)
  line L662 (1.3626, -4.7241) -> (0.6999, -5.4291)
  line L663 (0.6999, -5.4291) -> (0.0737, -6.2837)
  line L664 (0.0737, -6.2837) -> (0.0292, -7.3936)
  line L665 (-1.3538, -7.3436) -> (-0.1635, -8.1994)
  line L666 (-0.1635, -8.1994) -> (-0.029, -7.9915)
  line L667 (-0.029, -7.9915) -> (-0.0371, -7.3621)
  line L668 (-0.0371, -7.3621) -> (-0.1429, -6.3148)
  line L669 (-0.1429, -6.3148) -> (-0.578, -5.7009)
  line L670 (-0.578, -5.7009) -> (-1.089, -5.2488)
  line L671 (-1.089, -5.2488) -> (-1.7265, -5.3336)
  line L672 (-1.7265, -5.3336) -> (-2.3238, -5.5298)
  line L673 (-2.3238, -5.5298) -> (-2.5533, -5.8568)
  line L674 (-2.5533, -5.8568) -> (-2.6292, -6.0763)
  line L675 (-2.6292, -6.0763) -> (-2.5295, -6.3043)
  line L676 (-2.5295, -6.3043) -> (-1.3538, -7.3436)
  line L677 (5.9823, -7.3454) -> (6.3138, -8.6775)
  line L678 (6.3138, -8.6775) -> (6.581, -9.1553)
  line L679 (6.581, -9.1553) -> (6.9252, -8.8091)
  line L680 (6.9252, -8.8091) -> (7.4875, -7.6694)
  line L681 (7.4875, -7.6694) -> (8.3117, -5.8615)
  line L682 (8.3117, -5.8615) -> (8.3343, -5.4169)
  line L683 (8.3343, -5.4169) -> (8.1168, -5.1921)
  line L684 (8.1168, -5.1921) -> (7.2601, -4.9233)
  line L685 (7.2601, -4.9233) -> (6.3634, -4.7028)
  line L686 (6.3634, -4.7028) -> (5.8659, -4.8166)
  line L687 (5.8659, -4.8166) -> (5.6253, -4.9515)
  line L688 (5.6253, -4.9515) -> (5.5572, -5.2599)
  line L689 (5.5572, -5.2599) -> (5.9823, -7.3454)
  line L690 (-11.9403, -6.2414) -> (-11.6452, -6.8558)
  line L691 (-11.6452, -6.8558) -> (-10.9946, -7.3972)
  line L692 (-10.9946, -7.3972) -> (-10.296, -7.7817)
  line L693 (-10.296, -7.7817) -> (-9.6655, -7.2991)
  line L694 (-9.6655, -7.2991) -> (-9.1709, -6.6717)
  line L695 (-9.1709, -6.6717) -> (-9.4232, -6.0426)
  line L696 (-9.4232, -6.0426) -> (-9.6596, -5.6803)
  line L697 (-9.6596, -5.6803) -> (-9.9014, -5.5044)
  line L698 (-9.9014, -5.5044) -> (-10.9881, -5.514)
  line L699 (-10.9881, -5.514) -> (-11.9982, -5.6806)
  line L700 (-11.9982, -5.6806) -> (-12.0581, -5.8776)
  line L701 (-12.0581, -5.8776) -> (-11.9403, -6.2414)
  line L702 (10.2273, -8.2419) -> (10.3595, -9.2979)
  line L703 (10.3595, -9.2979) -> (10.6362, -9.8402)
  line L704 (10.6362, -9.8402) -> (11.2669, -10.04)
  line L705 (11.2669, -10.04) -> (12.4609, -10.0686)
  line L706 (12.4609, -10.0686) -> (14.264, -9.9656)
  line L707 (14.264, -9.9656) -> (14.4894, -9.7206)
  line L708 (14.4894, -9.7206) -> (14.5217, -9.2437)
  line L709 (14.5217, -9.2437) -> (14.4964, -8.7436)
  line L710 (14.4964, -8.7436) -> (14.3191, -8.3384)
  line L711 (14.3191, -8.3384) -> (12.9009, -6.9528)
  line L712 (12.9009, -6.9528) -> (11.3309, -5.7243)
  line L713 (11.3309, -5.7243) -> (10.9753, -5.7019)
  line L714 (10.9753, -5.7019) -> (10.621, -5.9487)
  line L715 (10.621, -5.9487) -> (10.2961, -6.247)
  line L716 (10.2961, -6.247) -> (10.1468, -6.5853)
  line L717 (10.1468, -6.5853) -> (10.2273, -8.2419)
  line L718 (6.4832, -9.937) -> (5.929, -7.4021)
  line L719 (5.929, -7.4021) -> (5.5846, -6.0311)
  line L720 (5.5846, -6.0311) -> (5.2662, -5.4469)
  line L721 (5.2662, -5.4469) -> (4.7907, -5.5354)
  line L722 (4.7907, -5.5354) -> (3.9747, -6.1821)
  line L723 (3.9747, -6.1821) -> (2.7042, -7.3867)
  line L724 (2.7042, -7.3867) -> (2.1884, -8.7172)
  line L725 (2.1884, -8.7172) -> (1.9994, -9.4984)
  line L726 (1.9994, -9.4984) -> (2.1395, -9.8996)
  line L727 (2.1395, -9.8996) -> (2.7917, -10.0474)
  line L728 (2.7917, -10.0474) -> (4.1388, -10.0685)
  line L729 (4.1388, -10.0685) -> (6.1873, -10.0521)
  line L730 (6.1873, -10.0521) -> (6.4832, -9.937)
  line L731 (10.1618, -8.2451) -> (9.9175, -6.6033)
  line L732 (9.9175, -6.6033) -> (9.6769, -6.2933)
  line L733 (9.6769, -6.2933) -> (9.2426, -6.0495)
  line L734 (9.2426, -6.0495) -> (8.7957, -5.8665)
  line L735 (8.7957, -5.8665) -> (8.4677, -5.982)
  line L736 (8.4677, -5.982) -> (7.5237, -7.7439)
  line L737 (7.5237, -7.7439) -> (6.9872, -9.0879)
  line L738 (6.9872, -9.0879) -> (6.9036, -9.778)
  line L739 (6.9036, -9.778) -> (7.3592, -10.0322)
  line L740 (7.3592, -10.0322) -> (8.4397, -10.0686)
  line L741 (8.4397, -10.0686) -> (9.5329, -10.0402)
  line L742 (9.5329, -10.0402) -> (10.0767, -9.8409)
  line L743 (10.0767, -9.8409) -> (10.2328, -9.2996)
  line L744 (10.2328, -9.2996) -> (10.1618, -8.2451)
  line L745 (-6.5419, -8.7085) -> (-6.374, -9.4948)
  line L746 (-6.374, -9.4948) -> (-6.1766, -9.8985)
  line L747 (-6.1766, -9.8985) -> (-5.8225, -10.0473)
  line L748 (-5.8225, -10.0473) -> (-5.1843, -10.0685)
  line L749 (-5.1843, -10.0685) -> (-4.5461, -10.0409)
  line L750 (-4.5461, -10.0409) -> (-4.1912, -9.848)
  line L751 (-4.1912, -9.848) -> (-3.9918, -9.3241)
  line L752 (-3.9918, -9.3241) -> (-3.8199, -8.304)
  line L753 (-3.8199, -8.304) -> (-3.6721, -6.7172)
  line L754 (-3.6721, -6.7172) -> (-3.8479, -6.4227)
  line L755 (-3.8479, -6.4227) -> (-4.2432, -6.1974)
  line L756 (-4.2432, -6.1974) -> (-4.6572, -6.0114)
  line L757 (-4.6572, -6.0114) -> (-4.9645, -5.9915)
  line L758 (-4.9645, -5.9915) -> (-5.8684, -6.602)
  line L759 (-5.8684, -6.602) -> (-6.4045, -7.0548)
  line L760 (-6.4045, -7.0548) -> (-6.6533, -7.4252)
  line L761 (-6.6533, -7.4252) -> (-6.6781, -7.9106)
  line L762 (-6.6781, -7.9106) -> (-6.5419, -8.7085)
  line L763 (-12.8865, -8.4761) -> (-11.9377, -7.0029)
  line L764 (-11.9377, -7.0029) -> (-11.8868, -6.6391)
  line L765 (-11.8868, -6.6391) -> (-12.0083, -6.2448)
  line L766 (-12.0083, -6.2448) -> (-12.1949, -5.8564)
  line L767 (-12.1949, -5.8564) -> (-12.4393, -5.6632)
  line L768 (-12.4393, -5.6632) -> (-13.7576, -5.6324)
  line L769 (-13.7576, -5.6324) -> (-14.6052, -5.7018)
  line L770 (-14.6052, -5.7018) -> (-15.0405, -5.9592)
  line L771 (-15.0405, -5.9592) -> (-15.2009, -6.6153)
  line L772 (-15.2009, -6.6153) -> (-15.2238, -7.8809)
  line L773 (-15.2238, -7.8809) -> (-15.1476, -9.7951)
  line L774 (-15.1476, -9.7951) -> (-14.9668, -10.0343)
  line L775 (-14.9668, -10.0343) -> (-14.6145, -10.0685)
  line L776 (-14.6145, -10.0685) -> (-14.2448, -10.0436)
  line L777 (-14.2448, -10.0436) -> (-13.9415, -9.8695)
  line L778 (-13.9415, -9.8695) -> (-12.8865, -8.4761)
  line L779 (0.3517, -9.321) -> (-0.1103, -8.5218)
  line L780 (-0.1103, -8.5218) -> (-1.3722, -7.4126)
  line L781 (-1.3722, -7.4126) -> (-2.6381, -6.4151)
  line L782 (-2.6381, -6.4151) -> (-2.8975, -6.3315)
  line L783 (-2.8975, -6.3315) -> (-3.1274, -6.3978)
  line L784 (-3.1274, -6.3978) -> (-3.3397, -6.5099)
  line L785 (-3.3397, -6.5099) -> (-3.4758, -6.746)
  line L786 (-3.4758, -6.746) -> (-3.7547, -8.3062)
  line L787 (-3.7547, -8.3062) -> (-3.8725, -9.3251)
  line L788 (-3.8725, -9.3251) -> (-3.6947, -9.8482)
  line L789 (-3.6947, -9.8482) -> (-3.0259, -10.041)
  line L790 (-3.0259, -10.041) -> (-1.6708, -10.0685)
  line L791 (-1.6708, -10.0685) -> (0.3454, -9.9752)
  line L792 (0.3454, -9.9752) -> (0.505, -9.7532)
  line L793 (0.505, -9.7532) -> (0.3517, -9.321)
  line L794 (-10.1929, -9.0251) -> (-10.1313, -9.6283)
  line L795 (-10.1313, -9.6283) -> (-9.9075, -9.9381)
  line L796 (-9.9075, -9.9381) -> (-9.3388, -10.0522)
  line L797 (-9.3388, -10.0522) -> (-8.2423, -10.0685)
  line L798 (-8.2423, -10.0685) -> (-7.1507, -10.0473)
  line L799 (-7.1507, -10.0473) -> (-6.6166, -9.8988)
  line L800 (-6.6166, -9.8988) -> (-6.4866, -9.4957)
  line L801 (-6.4866, -9.4957) -> (-6.6075, -8.7106)
  line L802 (-6.6075, -8.7106) -> (-6.8741, -7.4894)
  line L803 (-6.8741, -7.4894) -> (-7.178, -7.0884)
  line L804 (-7.178, -7.0884) -> (-7.5435, -6.85)
  line L805 (-7.5435, -6.85) -> (-8.2407, -6.7673)
  line L806 (-8.2407, -6.7673) -> (-8.9775, -6.797)
  line L807 (-8.9775, -6.797) -> (-9.6208, -7.3461)
  line L808 (-9.6208, -7.3461) -> (-10.163, -8.0327)
  line L809 (-10.163, -8.0327) -> (-10.1929, -9.0251)
  line L810 (-10.2577, -9.0273) -> (-10.3943, -8.0505)
  line L811 (-10.3943, -8.0505) -> (-11.0186, -7.4601)
  line L812 (-11.0186, -7.4601) -> (-11.4437, -7.1806)
  line L813 (-11.4437, -7.1806) -> (-11.7736, -7.1959)
  line L814 (-11.7736, -7.1959) -> (-12.8251, -8.5014)
  line L815 (-12.8251, -8.5014) -> (-13.4325, -9.4074)
  line L816 (-13.4325, -9.4074) -> (-13.5557, -9.8726)
  line L817 (-13.5557, -9.8726) -> (-13.1234, -10.044)
  line L818 (-13.1234, -10.044) -> (-12.0642, -10.0685)
  line L819 (-12.0642, -10.0685) -> (-10.9887, -10.0523)
  line L820 (-10.9887, -10.0523) -> (-10.442, -9.9384)
  line L821 (-10.442, -9.9384) -> (-10.2548, -9.6293)
  line L822 (-10.2548, -9.6293) -> (-10.2577, -9.0273)
  point P0 (0.8, -0.8588)
  constraints: 1646 end point, 20 parallel, 19 perpendicular
sketch "Sketch9" plane through (8.2638, 25.5, 2.7512) normal (1, 0, 0) x (0, 1, 0)
  line L0 (15.6267, 14.1538) -> (10.0956, 14.1587)
  line L1 (10.0956, 14.1587) -> (4.8594, 14.1635)
  line L2 (4.8594, 14.1635) -> (4.088, 14.1641)
  line L3 (4.088, 14.1641) -> (2.3563, 14.1657)
  line L4 (2.3563, 14.1657) -> (-2.257, 14.1698)
  line L5 (-2.257, 14.1698) -> (-3.8539, 14.1713)
  line L6 (-3.8539, 14.1713) -> (-7.4375, 14.1745)
  line L7 (-7.4375, 14.1745) -> (-15.1699, 14.1815)
  line L8 (-15.1699, 14.1815) -> (-15.2319, 14.1815)
  line L9 (-11.6818, 3.3732) -> (-12.0761, 2.933)
  line L10 (-10.7844, 10.3488) -> (-15.1699, 14.1815)
  line L11 (-10.7844, 10.3488) -> (-13.8452, 7.5417)
  line L12 (-10.5757, 10.321) -> (-10.7844, 10.3488)
  line L13 (-10.9642, 6.6282) -> (-13.8452, 7.5417)
  line L14 (-10.9642, 6.6282) -> (-11.6818, 3.3732)
  line L15 (-9.678, -1.5748) -> (-9.9814, -1.1521)
  line L16 (-9.2499, 7.1724) -> (-10.9642, 6.6282)
  line L17 (-9.2003, 7.1521) -> (-9.2499, 7.1724)
  line L18 (-9.925, 1.4399) -> (-12.0761, 2.933)
  line L19 (-9.2499, 7.1724) -> (-10.5757, 10.321)
  line L20 (-9.925, 1.4399) -> (-9.9814, -1.1521)
  line L21 (-7.7475, 12.6014) -> (-7.4375, 14.1745)
  line L22 (-7.7475, 12.6014) -> (-10.5757, 10.321)
  line L23 (-9.2122, 4.3116) -> (-11.6818, 3.3732)
  line L24 (-9.2122, 4.3116) -> (-9.2003, 7.1521)
  line L25 (-7.2029, 7.4306) -> (-9.2003, 7.1521)
  line L26 (-7.2262, 2.5933) -> (-9.925, 1.4399)
  line L27 (-7.2262, 2.5933) -> (-9.2122, 4.3116)
  line L28 (-6.7305, 2.5195) -> (-7.2262, 2.5933)
  line L29 (-6.5189, 8.0514) -> (-7.2029, 7.4306)
  line L30 (-5.8401, -0.535) -> (-9.678, -1.5748)
  line L31 (-5.3398, 0.4698) -> (-5.8401, -0.535)
  line L32 (-5.3398, 0.4698) -> (-6.7305, 2.5195)
  line L33 (-6.3417, 9.2804) -> (-6.5189, 8.0514)
  line L34 (-6.3417, 9.2804) -> (-7.7475, 12.6014)
  line L35 (-6.352, 3.752) -> (-6.7305, 2.5195)
  line L36 (-6.352, 3.752) -> (-7.2029, 7.4306)
  line L37 (-3.3195, 0.7918) -> (-5.3398, 0.4698)
  line L38 (-3.5356, 6.7166) -> (-6.5189, 8.0514)
  line L39 (-3.5226, 6.6987) -> (-3.5356, 6.7166)
  line L40 (-3.7408, 5.385) -> (-6.352, 3.752)
  line L41 (-3.7408, 5.385) -> (-3.5226, 6.6987)
  line L42 (-3.477, 10.4478) -> (-6.3417, 9.2804)
  line L43 (-3.477, 10.4478) -> (-3.8539, 14.1713)
  line L44 (-2.1303, 1.9717) -> (-3.3195, 0.7918)
  line L45 (-2.0839, 2.4881) -> (-2.1303, 1.9717)
  line L46 (-2.7188, 9.871) -> (-3.477, 10.4478)
  line L47 (-2.0839, 2.4881) -> (-3.7408, 5.385)
  line L48 (-2.5276, 9.8784) -> (-2.7188, 9.871)
  line L49 (-2.7188, 9.871) -> (-3.5356, 6.7166)
  line L50 (-2.0106, 6.673) -> (-3.5226, 6.6987)
  line L51 (-0.9613, 9.0998) -> (-2.5276, 9.8784)
  line L52 (-1.0697, 11.6538) -> (-2.257, 14.1698)
  line L53 (-1.0697, 11.6538) -> (-2.5276, 9.8784)
  line L54 (-0.2079, 5.212) -> (-2.0106, 6.673)
  line L55 (-0.2079, 5.212) -> (-2.0839, 2.4881)
  line L56 (-0.7595, 8.4985) -> (-0.9613, 9.0998)
  line L57 (-0.7595, 8.4985) -> (-2.0106, 6.673)
  line L58 (0.1704, 5.3001) -> (-0.2079, 5.212)
  line L59 (0.0555, 11.2063) -> (-1.0697, 11.6538)
  line L60 (0.2384, 10.4521) -> (-0.9613, 9.0998)
  line L61 (0.2384, 10.4521) -> (0.0555, 11.2063)
  line L62 (2.7149, 0.8141) -> (-2.1303, 1.9717)
  line L63 (1.4518, 7.3795) -> (-0.7595, 8.4985)
  line L64 (2.868, 0.1938) -> (2.7149, 0.8141)
  line L65 (1.4518, 7.3795) -> (0.1704, 5.3001)
  line L66 (0.0555, 11.2063) -> (2.3563, 14.1657)
  line L67 (3.1852, 2.3794) -> (2.7149, 0.8141)
  line L68 (2.8096, 8.0422) -> (1.4518, 7.3795)
  line L69 (3.1602, 2.5218) -> (3.1852, 2.3794)
  line L70 (3.1602, 2.5218) -> (0.1704, 5.3001)
  line L71 (2.5801, 9.2559) -> (0.2384, 10.4521)
  line L72 (2.5801, 9.2559) -> (2.8096, 8.0422)
  line L73 (3.9123, 7.3853) -> (2.8096, 8.0422)
  line L74 (2.5801, 9.2559) -> (4.088, 14.1641)
  line L75 (4.2913, 6.4296) -> (3.9123, 7.3853)
  line L76 (4.2913, 6.4296) -> (3.1602, 2.5218)
  line L77 (6.412, 9.282) -> (3.9123, 7.3853)
  line L78 (6.4294, 9.2776) -> (6.412, 9.282)
  line L79 (6.4149, 9.2729) -> (4.8594, 14.1635)
  line L80 (6.8569, 5.534) -> (4.2913, 6.4296)
  line L81 (7.3482, 3.1538) -> (3.1852, 2.3794)
  line L82 (7.3482, 3.1538) -> (6.8569, 5.534)
  line L83 (7.7155, 0.1558) -> (2.868, 0.1938)
  line L84 (9.5528, 1.5223) -> (7.3482, 3.1538)
  line L85 (9.5528, 1.5223) -> (7.7155, 0.1558)
  line L86 (9.6495, 1.52) -> (9.5528, 1.5223)
  line L87 (7.8984, 6.4684) -> (6.8569, 5.534)
  line L88 (7.8838, 6.4638) -> (6.4149, 9.2729)
  line L89 (8.3371, 9.6656) -> (6.4297, 9.276)
  line L90 (10.1933, 12.4785) -> (10.0956, 14.1587)
  line L91 (10.1787, 12.4738) -> (8.3371, 9.6656)
  line L92 (9.4798, 6.7649) -> (7.8838, 6.4638)
  line L93 (9.6575, 7.3124) -> (9.4943, 6.7695)
  line L94 (9.6575, 7.3124) -> (8.3517, 9.6702)
  line L95 (11.2205, 3.8998) -> (9.6495, 1.52)
  line L96 (11.2224, 3.9754) -> (11.2205, 3.8998)
  line L97 (11.2079, 3.9708) -> (9.4798, 6.7649)
  line L98 (11.422, 8.6705) -> (9.6575, 7.3124)
  line L99 (11.8053, 9.7292) -> (10.1787, 12.4738)
  line L100 (11.8053, 9.7292) -> (11.4075, 8.6659)
  line L101 (13.0152, 6.2418) -> (11.2079, 3.9708)
  line L102 (13.0152, 6.2418) -> (11.4075, 8.6659)
  line L103 (13.3289, 9.642) -> (11.8199, 9.7338)
  line L104 (16.1386, 7.3478) -> (13.0297, 6.2465)
  line L105 (16.1386, 7.3478) -> (13.3289, 9.642)
  line L106 (13.3289, 9.642) -> (15.6267, 14.1538)
  point P0 (-25.5, -2.7512)
  point P1 (3.1602, 2.5218)
  point P2 (-6.352, 3.752)
  point P3 (-6.7305, 2.5195)
  point P4 (3.1852, 2.3794)
  point P5 (4.8594, 14.1635)
  point P6 (2.8096, 8.0422)
  point P7 (3.9123, 7.3853)
  point P8 (6.412, 9.282)
  constraints: 214 end point, 1 point on line